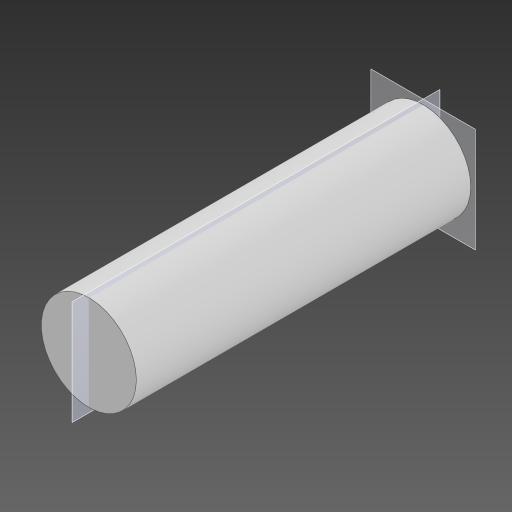
# Autodesk Inventor part: UpperArmActuatorShaftBoundingBox
Saved by Autodesk Inventor 2023 (Build 270158000, 158)
## iProperties
Created: 2023-03-24
Part Number: UpperArmActuatorShaftBoundingBox
Material: Generic
Document SubType Name: Modeling
Designer: Val
Density: 1 g/cm^3
Appearance: Default
Author: Val
Autodesk Inventor part; units mm, degrees
ref_plane "XZ Plane" through (0, 0, 0) normal (0, 1, 0) x (-1, 0, 0)
sketch "Sketch1" plane through (0, 0, 0) normal (0, 0, 1) x (1, 0, 0)
  circle A0 centre (0, 0) radius 9.525 projected
  point P0 (0, 0)
  dimension "d0" = 67
extrude "Extrusion1" add sketch "Sketch1" along normal blind 67
body "Solid1"
